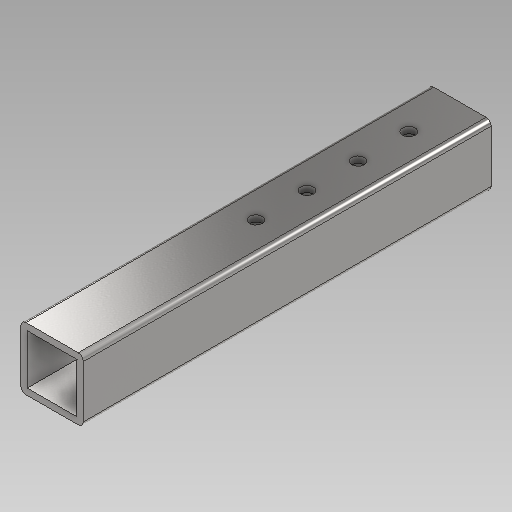
# Autodesk Inventor part: member_vertical_inner
Saved by Autodesk Inventor 2021 (Build 250183000, 183)
## iProperties
Created: 2021-06-01
Part Number: member_vertical_inner
Material: Steel, Galvanized
Document SubType Name: Modeling
Designer: Watchdog
Density: 7.85 g/cm^3
Appearance: Galvanized
Author: Watchdog
Autodesk Inventor part; units mm, degrees
ref_plane "YZ Plane" through (0, 0, 0) normal (1, 0, 0) x (0, 1, 0)
ref_plane "XZ Plane" through (0, 0, 0) normal (0, 1, 0) x (-1, 0, 0)
ref_plane "XY Plane" through (0, 0, 0) normal (0, 0, 1) x (1, 0, 0)
sketch "Sketch1" plane through (0, 0, 0) normal (0, 0, 1) x (1, 0, 0)
  line L0 (-12.25, 12.25) -> (12.25, 12.25)
  line L1 (12.25, 12.25) -> (12.25, -12.25)
  line L2 (12.25, -12.25) -> (-12.25, -12.25)
  line L3 (-12.25, -12.25) -> (-12.25, 12.25)
  line L4 (9.75, 9.75) -> (-9.75, 9.75)
  line L5 (-9.75, 9.75) -> (-9.75, -9.75)
  line L6 (-9.75, -9.75) -> (9.75, -9.75)
  line L7 (9.75, -9.75) -> (9.75, 9.75)
  point P0 (0, 0)
  dimension "d0" = 24.5
  dimension "d1" = 24.5
  dimension "d2" = 12.25
  dimension "d3" = 12.25
  dimension "d4" = 2.5
  constraints: 16 end point, 4 parallel, 2 perpendicular, 1 horizontal, 3 other
  measures "d0" distance of L0.start L0.end
  measures "d1" distance of L2.end L0.start
  measures "d2" distance from line of point (0, 0) L0
  measures "d3" distance from line of point (0, 0) L3
  measures "d4" distance between parallel lines of L0 L4
extrude "Extrusion1" add sketch "Sketch1" along normal blind 1000
fillet "Fillet1" radius 2 4 edges at (12.25, 12.25, 500) (-12.25, 12.25, 500) (-12.25, -12.25, 500) (12.25, -12.25, 500)
ref_plane "Work Plane1" through (0, 0, 160) normal (0, 0, -1) x (-1, 0, 0)
split "Split1" plane through (0, 0, 160) removes the side toward (0, 0, 1)
sketch "Sketch2" plane through (-10.25, 12.25, 0) normal (0, 1, 0) x (1, 0, 0)
  point P0 (10.25, 0)
  point P1 (10.25, -20)
  dimension "d9" = 0
  dimension "d10" = 20
  measures "d9" horizontal distance of point (10.25, 0) point (10.25, -20)
  measures "d10" distance of point (10.25, 0) point (10.25, -20)
hole "Hole1" at (0, 12.25, 20) direction (0, -1, 0) diameter 5 end through all
pattern_linear "Rectangular Pattern1" count 4 spacing 20 along (0, 0, 1) of "Hole1"
equation "\"d0\" = -2 * a + sm_varx_squareBarDimension - tol"
equation "\"d1\" = d0"
equation "\"d2\" = 0.5 * d1"
equation "\"d3\" = 0.5 * d0"
equation "\"d4\" = a"
equation "\"d10\" = 0.666667 * sm_varx_squareBarDimension"
equation "\"d11\" = sm_varx_pinPlate_holeDiameter"
equation "\"d20\" = 0.666667 * sm_varx_squareBarDimension"
equation "\"sm_varx_squareBarThickness\" = 2.5"
equation "\"sm_varx_pinPlate_holeDiameter\" = 5"
equation "\"a\" = sm_varx_squareBarThickness"
equation "\"tol\" = sm_varx_member_tolerance"
equation "\"sm_varx_member_tolerance\" = 0.5"
equation "\"hoop_angle_z\" = 45deg"
equation "\"hoop_bearing_length\" = 5deg"
equation "\"hoop_cable_diam\" = 5"
equation "\"hoop_cable_pulley_diam\" = 22"
equation "\"rack_tooth_addendum\" = 5"
equation "\"rack_tooth_dedendum\" = 5"
equation "\"rack_tooth_thickness\" = 5"
equation "\"secure_arm_angle\" = 20deg"
equation "\"secure_arm_hold_length\" = 35"
equation "\"secure_arm_radii\" = 9"
equation "\"support_baseClamp_platformLengthBuffer\" = 35"
equation "\"support_baseClamp_platformThickness\" = 15"
equation "\"support_baseClamp_platformWidthBuffer\" = 0"
equation "\"support_baseClamp_sleeveHoleDiameter\" = 12"
equation "\"support_baseClamp_sleeveSweepTerminationAngle\" = 55deg"
equation "\"support_baseClamp_thickness\" = 8"
equation "\"support_frame_endHoleBuffer\" = 25"
equation "\"support_frame_squareBarFillet\" = 2"
equation "\"support_frame_squareBarThickness\" = 5"
equation "\"hoop_tabs_thickness\" = 6"
equation "\"hoop_tabs_hole\" = 4"
equation "\"wheelchair_deployed_width\" = 635"
equation "\"wheelchair_deployed_length\" = 1067"
equation "\"wheelchair_deployed_height\" = 914"
equation "\"sm_varx_pinPlate_thickness\" = 5"
equation "\"sm_varx_squareBarDimension\" = 30"
body "Solid1"
